Autodesk Fusion 360 part; units mm, degrees
(part 2 of 2)
sketch "Sketch31" plane through (0, 0, 7) normal (0, 0, 1) x (1, 0, 0)
  line L0 (-163.65, 58) -> (-174.35, 58)
  line L1 (-174.35, 58) -> (-174.35, 48)
  line L2 (-174.35, 48) -> (-163.65, 48)
  line L3 (-163.65, 48) -> (-163.65, 58)
  line L4 (-169, 58) -> (-169, 53)
  circle A0 centre (-169, 53) radius 2.35
  dimension "d256" = 5
  dimension "d257" = 4.7
  constraint midpoint L0 L4.start
  constraint perpendicular L0 L4
  constraint coincident L4.end A0.centre
  measures "d256" distance of L4.start L4.end
  measures "d257" diameter of A0
extrude "Extrude70" cut sketch "Sketch31" against normal blind 20.5 contours A0 bodies 5 8
sketch "Sketch32" plane through (0, 58, 0) normal (0, 1, 0) x (-1, 0, 0)
  line L0 (174.35, 10.3) -> (174.35, 7)
  line L1 (174.35, 7) -> (163.65, 7)
  line L2 (163.65, 7) -> (163.65, 10.3)
  line L3 (163.65, 10.3) -> (174.35, 10.3)
  line L4 (181.65, 4) -> (183.5, 4)
  line L5 (183.5, 4) -> (183.5, 13)
  line L6 (183.5, 13) -> (137, 13)
  line L7 (137, 13) -> (137, 4)
  line L8 (137, 4) -> (138.85, 4)
  arc A0 (147.15, 4) -> (138.85, 4) centre (143, 4) ccw
  line L9 (147.15, 4) -> (156.1, 4)
  arc A1 (164.4, 4) -> (156.1, 4) centre (160.25, 4) ccw
  line L10 (164.4, 4) -> (173.35, 4)
  arc A2 (181.65, 4) -> (173.35, 4) centre (177.5, 4) ccw
  line L11 (151.625, 4) -> (151.625, 7)
  line L12 (151.625, 7) -> (156.975, 7)
  line L13 (156.975, 7) -> (156.975, 10.3)
  line L14 (156.975, 10.3) -> (151.625, 10.3)
  line L15 (151.625, 10.3) -> (151.625, 7)
  line L16 (151.625, 7) -> (146.275, 7)
  line L17 (146.275, 7) -> (146.275, 10.3)
  line L18 (146.275, 10.3) -> (151.625, 10.3)
  line L19 (151.625, 10.3) -> (151.625, 7)
  dimension "d260" = 3
  dimension "d261" = 3.3
  dimension "d262" = 5.35
  dimension "d263" = 3.3
  constraint midpoint L9 L11.start
  constraint perpendicular L9 L11
  constraint horizontal L12
  constraint vertical L13
  constraint horizontal L14
  constraint vertical L15
  constraint horizontal L16
  constraint vertical L17
  constraint horizontal L18
  constraint vertical L19
  measures "d260" distance of L11.start L11.end
  measures "d261" distance of L11.end L14.end
  measures "d262" distance of L11.end L12.end
  measures "d263" distance of L11.end L14.end
extrude "Extrude71" cut sketch "Sketch32" against normal blind 10 contours L12 L13 L14 L15 L19 | L15 L16 L17 L18 L19 bodies 5
sketch "Sketch33" plane through (0, 0, 7) normal (0, 0, 1) x (1, 0, 0)
  line L0 (-146.275, 58) -> (-156.975, 58)
  line L1 (-156.975, 58) -> (-156.975, 48)
  line L2 (-156.975, 48) -> (-146.275, 48)
  line L3 (-146.275, 48) -> (-146.275, 58)
  line L4 (-151.625, 58) -> (-151.625, 53)
  circle A0 centre (-151.625, 53) radius 2.35
  dimension "d266" = 5
  dimension "d267" = 4.7
  constraint midpoint L0 L4.start
  constraint perpendicular L0 L4
  constraint coincident L4.end A0.centre
  measures "d266" distance of L4.start L4.end
  measures "d267" diameter of A0
extrude "Extrude72" cut sketch "Sketch33" against normal blind 21 contours A0 bodies 5 8
sketch "Sketch34" plane through (0, 29, 0) normal (0, -1, 0) x (1, 0, 0)
  line L0 (-183.5, 4) -> (-181.65, 4)
  arc A0 (-173.35, 4) -> (-181.65, 4) centre (-177.5, 4) ccw
  line L1 (-173.35, 4) -> (-164.4, 4)
  arc A1 (-156.1, 4) -> (-164.4, 4) centre (-160.25, 4) ccw
  line L2 (-156.1, 4) -> (-147.15, 4)
  arc A2 (-138.85, 4) -> (-147.15, 4) centre (-143, 4) ccw
  line L3 (-138.85, 4) -> (-137, 4)
  line L4 (-137, 4) -> (-137, 13)
  line L5 (-137, 13) -> (-183.5, 13)
  line L6 (-183.5, 13) -> (-183.5, 4)
  line L7 (-151.625, 4) -> (-151.625, 7)
  line L8 (-168.875, 4) -> (-168.875, 7)
  line L9 (-168.875, 7) -> (-163.525, 7)
  line L10 (-163.525, 7) -> (-163.525, 10.3)
  line L11 (-163.525, 10.3) -> (-168.875, 10.3)
  line L12 (-168.875, 10.3) -> (-168.875, 7)
  line L13 (-151.625, 7) -> (-156.975, 7)
  line L14 (-156.975, 7) -> (-156.975, 10.3)
  line L15 (-156.975, 10.3) -> (-151.625, 10.3)
  line L16 (-151.625, 10.3) -> (-151.625, 7)
  line L17 (-151.625, 7) -> (-146.275, 7)
  line L18 (-146.275, 7) -> (-146.275, 10.3)
  line L19 (-146.275, 10.3) -> (-151.625, 10.3)
  line L20 (-151.625, 10.3) -> (-151.625, 7)
  line L21 (-168.875, 10.3) -> (-174.225, 10.3)
  line L22 (-174.225, 10.3) -> (-174.225, 7)
  line L23 (-174.225, 7) -> (-168.875, 7)
  line L24 (-168.875, 7) -> (-168.875, 10.3)
  dimension "d270" = 3
  dimension "d271" = 3
  dimension "d272" = 3.3
  dimension "d273" = 5.35
  dimension "d274" = 5.35
  dimension "d275" = 3.3
  dimension "d276" = 5.35
  dimension "d277" = 5.35
  constraint midpoint L2 L7.start
  constraint perpendicular L2 L7
  constraint midpoint L1 L8.start
  constraint perpendicular L1 L8
  constraint horizontal L9
  constraint vertical L10
  constraint horizontal L11
  constraint vertical L12
  constraint horizontal L13
  constraint vertical L14
  constraint horizontal L15
  constraint vertical L16
  constraint horizontal L17
  constraint vertical L18
  constraint horizontal L19
  constraint vertical L20
  constraint horizontal L21
  constraint vertical L22
  constraint horizontal L23
  constraint vertical L24
  measures "d270" distance of L7.start L7.end
  measures "d271" distance of L8.start L8.end
  measures "d272" distance of L8.end L11.end
  measures "d273" distance of L8.end L9.end
  measures "d274" distance of L7.end L13.end
  measures "d275" distance of L7.end L15.end
  measures "d276" distance of L7.end L17.end
  measures "d277" distance of L11.end L21.end
extrude "Extrude73" cut sketch "Sketch34" against normal blind 10 contours L9 L10 L11 L12 L24 | L12 L21 L22 L23 L24 | L13 L14 L15 L16 L20 | L16 L17 L18 L19 L20 bodies 5
sketch "Sketch35" plane through (0, 0, 7) normal (0, 0, 1) x (1, 0, 0)
  line L0 (-156.975, 29) -> (-146.275, 29)
  line L1 (-146.275, 29) -> (-146.275, 39)
  line L2 (-146.275, 39) -> (-156.975, 39)
  line L3 (-156.975, 39) -> (-156.975, 29)
  line L4 (-151.625, 29) -> (-151.625, 34)
  circle A0 centre (-151.625, 34) radius 2.35
  dimension "d280" = 5
  dimension "d281" = 4.7
  constraint midpoint L0 L4.start
  constraint perpendicular L0 L4
  constraint coincident L4.end A0.centre
  measures "d280" distance of L4.start L4.end
  measures "d281" diameter of A0
extrude "Extrude74" cut sketch "Sketch35" against normal blind 20 contours A0 bodies 5 8
sketch "Sketch36" plane through (0, 0, 7) normal (0, 0, 1) x (1, 0, 0)
  line L0 (-174.225, 29) -> (-163.525, 29)
  line L1 (-163.525, 29) -> (-163.525, 39)
  line L2 (-163.525, 39) -> (-174.225, 39)
  line L3 (-174.225, 39) -> (-174.225, 29)
  line L4 (-168.875, 29) -> (-168.875, 34)
  circle A0 centre (-168.875, 34) radius 2.35
  dimension "d284" = 5
  dimension "d285" = 4.7
  constraint midpoint L0 L4.start
  constraint perpendicular L0 L4
  constraint coincident L4.end A0.centre
  measures "d284" distance of L4.start L4.end
  measures "d285" diameter of A0
extrude "Extrude75" cut sketch "Sketch36" against normal blind 23 contours A0 bodies 5 8
chamfer "Chamfer9" distance 2.5 angle 45 1 edges at (-163.525, 39, 8.65) on bodies 5
chamfer "Chamfer10" distance 2.5 angle 45 1 edges at (-174.225, 39, 8.65) on bodies 5
chamfer "Chamfer11" distance 2.5 angle 45 1 edges at (-146.275, 39, 8.65) on bodies 5
chamfer "Chamfer12" distance 2.5 angle 45 1 edges at (-156.975, 39, 8.65) on bodies 5
chamfer "Chamfer13" distance 2.5 angle 45 1 edges at (-146.275, 48, 8.65) on bodies 5
chamfer "Chamfer14" distance 2.5 angle 45 1 edges at (-163.65, 48, 8.65) on bodies 5
chamfer "Chamfer15" distance 2.5 angle 45 1 edges at (-156.975, 48, 8.65) on bodies 5
chamfer "Chamfer16" distance 2.5 angle 45 1 edges at (-174.35, 48, 8.65) on bodies 5
